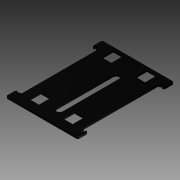
# Autodesk Inventor part: BED ROD MOUNT
Saved by Autodesk Inventor 2013 (Build 170138000, 138)
## iProperties
Created: 2014-03-03
Part Number: BED ROD MOUNT
Material: Generic
Document SubType Name: Modeling
Designer: employee
Density: 1 g/cm^3
Author: employee
Autodesk Inventor part; units mm, degrees
ref_plane "YZ Plane" through (0, 0, 0) normal (1, 0, 0) x (0, 1, 0)
ref_plane "XZ Plane" through (0, 0, 0) normal (0, 1, 0) x (-1, 0, 0)
ref_plane "XY Plane" through (0, 0, 0) normal (0, 0, 1) x (1, 0, 0)
sketch "Sketch1" plane through (0, 0, 0) normal (0, 0, 1) x (1, 0, 0)
  line L0 (-127, 170) -> (127, 170)
  line L1 (127, 170) -> (127, -170)
  line L2 (127, -170) -> (-127, -170)
  line L3 (-127, -170) -> (-127, 170)
  point P0 (0, 0)
  point P1 (0, 170)
  point P2 (-127, 0)
  dimension "d0" = 340
  dimension "d2" = 254
  constraints: 8 end point, 2 midpoint, 2 parallel, 1 horizontal, 1 horizontal alignment, 1 perpendicular, 1 vertical alignment
  measures "d0" distance of L2.end L0.start
  measures "d2" distance of L0.start L0.end
extrude "Extrusion1" add sketch "Sketch1" along normal blind 6.477
sketch "Sketch2" plane through (0, 0, 6.477) normal (0, 0, 1) x (1, 0, 0)
  line L0 (-127, 170) -> (-127, -170) projected
  line L1 (-127, 135) -> (-107, 135)
  line L2 (-107, 135) -> (-107, -135)
  line L3 (-107, -135) -> (-127, -135)
  line L4 (-127, -135) -> (-127, 135)
  point P0 (0, 0)
  point P1 (-127, 0)
  point P2 (-127, 0)
  dimension "d5" = 270
  dimension "d7" = 20
  constraints: 8 end point, 2 midpoint, 2 parallel, 1 coincident, 1 horizontal, 1 perpendicular, 1 point on line
  measures "d5" distance of L1.end L2.end
  measures "d7" distance of L1.start L1.end
extrude "Extrusion2" cut sketch "Sketch2" against normal through all
sketch "Sketch3" plane through (0, 0, 6.477) normal (0, 0, 1) x (1, 0, 0)
  line L0 (-127, 135) -> (-107, 135) projected
  line L1 (-119.8284, 135) -> (-114.1716, 135)
  line L2 (-114.1716, 135) -> (-114.1716, 145)
  line L3 (-114.1716, 145) -> (-119.8284, 145)
  line L4 (-119.8284, 145) -> (-119.8284, 135)
  circle A0 centre (-117, 145) radius 4
  line L5 (-117, 145) -> (-119.8284, 147.8284)
  point P0 (0, 0)
  point P1 (-117, 135)
  point P2 (-117, 135)
  point P3 (-117, 135)
  dimension "d14" = 8
  dimension "d10" = 10
  dimension "d12" = 135
  constraints: 10 end point, 4 midpoint, 2 parallel, 1 coincident, 1 horizontal, 1 perpendicular, 1 point on line, 1 vertical alignment, 3 other
  measures "d10" distance of L3.end L1.start
  measures "d12" angle of L5 L3
extrude "Extrusion3" cut sketch "Sketch3" against normal through all contours L4 A0 L2 L0 | L4 L3 L2 A0
sketch "Sketch4" plane through (0, 0, 6.477) normal (0, 0, 1) x (1, 0, 0)
  line L0 (-119.8284, 135) -> (-119.8284, 145) projected
  line L1 (-119.8284, 145) -> (-114.1716, 145) projected
  line L2 (-121, 142) -> (-113, 142)
  line L3 (-113, 142) -> (-113, 138)
  line L4 (-113, 138) -> (-121, 138)
  line L5 (-121, 138) -> (-121, 142)
  line L6 (-113, 142) -> (-112, 142)
  line L7 (-112, 142) -> (-112, 138)
  line L8 (-112, 138) -> (-113, 138)
  line L9 (-113, 138) -> (-113, 142)
  line L10 (-121, 142) -> (-122, 142)
  line L11 (-122, 142) -> (-122, 138)
  line L12 (-122, 138) -> (-121, 138)
  line L13 (-121, 138) -> (-121, 142)
  point P0 (0, 0)
  point P1 (-117, 142)
  point P2 (-117, 145)
  point P3 (-121, 140)
  point P4 (-119.8284, 140)
  dimension "d17" = 4
  dimension "d19" = 8
  dimension "d20" = 1
  constraints: 24 end point, 6 parallel, 4 midpoint, 3 horizontal, 3 perpendicular, 1 collinear, 1 horizontal alignment, 1 vertical alignment
  measures "d17" distance of L6.end L7.end
  measures "d19" distance between parallel lines of L3 L5
  measures "d20" distance of L2.end L6.end
extrude "Extrusion4" cut sketch "Sketch4" against normal through all contours L3 L6 L7 L8 | L12 L11 L10 L5
fillet "Fillet1" radius 5 2 edges at (-127, 170, 3.2385) (-127, 135, 3.2385)
fillet "Fillet1" radius 2.5 1 edges at (-107, 135, 3.2385)
mirror "Mirror1" about plane through (0, 0, 0) normal (1, 0, 0) of "Extrusion2"
mirror "Mirror2" about plane through (0, 0, 0) normal (1, 0, 0) of "Extrusion4", "Extrusion3", "Fillet1"
mirror "Mirror3" about plane through (0, 0, 0) normal (0, 1, 0) of "Extrusion4", "Extrusion3", "Fillet1", "Mirror2"
sketch "Sketch5" plane through (0, 0, 6.477) normal (0, 0, 1) x (1, 0, 0)
  line L0 (-109.5, -135) -> (-114.1716, -135) projected
  line L1 (-113, 142) -> (-112, 142) projected
  line L2 (20.5, -116.5) -> (20.5, 83.5)
  arc A0 (20.5, 83.5) -> (-1.5, 83.5) centre (9.5, 83.5) ccw
  line L3 (-1.5, 83.5) -> (-1.5, -116.5)
  arc A1 (-1.5, -116.5) -> (20.5, -116.5) centre (9.5, -116.5) ccw
  point P0 (0, 0)
  dimension "d31" = 18.5
  dimension "d32" = 11
  dimension "d33" = 200
  dimension "d34" = 9.5
  constraints: 4 end point, 4 point on circle, 4 tangent, 2 centre point, 1 parallel, 1 perpendicular
  measures "d31" distance from line of A1.centre L0
  measures "d32" radius of A1
  measures "d33" distance of L2.start L2.end
  measures "d34" horizontal distance of A1.centre point (0, 0)
extrude "Extrusion5" cut sketch "Sketch5" against normal through all
sketch "Sketch6" plane through (0, 0, 0) normal (0, 0, -1) x (-1, 0, 0)
  line L0 (-42, 159.6) -> (-77, 159.6) projected
  line L1 (-77, 159.6) -> (-77, 137.6) projected
  line L2 (-77, 137.6) -> (-42, 137.6) projected
  line L3 (-42, 137.6) -> (-42, 159.6) projected
  line L4 (42, -138.4) -> (77, -138.4) projected
  line L5 (77, -138.4) -> (77, -116.4) projected
  line L6 (77, -116.4) -> (42, -116.4) projected
  line L7 (42, -116.4) -> (42, -138.4) projected
  line L8 (-42, -138.4) -> (-42, -116.4) projected
  line L9 (-42, -116.4) -> (-77, -116.4) projected
  line L10 (-77, -116.4) -> (-77, -138.4) projected
  line L11 (-77, -138.4) -> (-42, -138.4) projected
  line L12 (42, 159.6) -> (42, 137.6) projected
  line L13 (42, 137.6) -> (77, 137.6) projected
  line L14 (77, 137.6) -> (77, 159.6) projected
  line L15 (77, 159.6) -> (42, 159.6) projected
  line L16 (101.6, -91) -> (101.6, 112.2) projected
  line L17 (-9.525, 112.2) -> (-101.6, 112.2) projected
  line L18 (-101.6, 112.2) -> (-101.6, -91) projected
  line L19 (-101.6, -91) -> (101.6, -91) projected
  line L20 (112, 138) -> (113, 138) projected
  line L21 (113, 138) -> (113, 142) projected
  line L22 (113, 142) -> (112, 142) projected
  line L23 (112, 142) -> (112, 138) projected
  line L24 (122, 142) -> (121, 142) projected
  line L25 (121, 142) -> (121, 138) projected
  line L26 (121, 138) -> (122, 138) projected
  line L27 (122, 138) -> (122, 142) projected
  line L28 (-121, 142) -> (-122, 142) projected
  line L29 (-122, 142) -> (-122, 138) projected
  line L30 (-122, 138) -> (-121, 138) projected
  line L31 (-121, 138) -> (-121, 142) projected
  line L32 (-113, 142) -> (-113, 138) projected
  line L33 (-113, 138) -> (-112, 138) projected
  line L34 (-112, 138) -> (-112, 142) projected
  line L35 (-112, 142) -> (-113, 142) projected
  line L36 (121, -142) -> (122, -142) projected
  line L37 (122, -142) -> (122, -138) projected
  line L38 (122, -138) -> (121, -138) projected
  line L39 (121, -138) -> (121, -142) projected
  line L40 (113, -142) -> (113, -138) projected
  line L41 (113, -138) -> (112, -138) projected
  line L42 (112, -138) -> (112, -142) projected
  line L43 (112, -142) -> (113, -142) projected
  line L44 (-121, -138) -> (-122, -138) projected
  line L45 (-122, -138) -> (-122, -142) projected
  line L46 (-122, -142) -> (-121, -142) projected
  line L47 (-121, -142) -> (-121, -138) projected
  line L48 (-112, -142) -> (-112, -138) projected
  line L49 (-112, -138) -> (-113, -138) projected
  line L50 (-113, -138) -> (-113, -142) projected
  line L51 (-113, -142) -> (-112, -142) projected
  line L52 (-127, -165) -> (-127, 165) projected
  arc A0 (-122, 170) -> (-127, 165) centre (-122, 165) ccw projected
  line L53 (-122, 170) -> (122, 170) projected
  arc A1 (127, 165) -> (122, 170) centre (122, 165) ccw projected
  line L54 (127, 165) -> (127, -165) projected
  arc A2 (122, -170) -> (127, -165) centre (122, -165) ccw projected
  line L55 (122, -170) -> (-122, -170) projected
  arc A3 (-127, -165) -> (-122, -170) centre (-122, -165) ccw projected
  line L56 (-77, -116.4) -> (-42, -116.4)
  line L57 (-42, -116.4) -> (-42, -96.4)
  line L58 (-42, -96.4) -> (-77, -96.4)
  line L59 (-77, -96.4) -> (-77, -116.4)
  line L60 (42, -116.4) -> (77, -116.4)
  line L61 (77, -116.4) -> (77, -96.4)
  line L62 (77, -96.4) -> (42, -96.4)
  line L63 (42, -96.4) -> (42, -116.4)
  line L64 (-77, 137.6) -> (-42, 137.6)
  line L65 (-42, 137.6) -> (-42, 117.6)
  line L66 (-42, 117.6) -> (-77, 117.6)
  line L67 (-77, 117.6) -> (-77, 137.6)
  line L68 (42, 137.6) -> (77, 137.6)
  line L69 (77, 137.6) -> (77, 117.6)
  line L70 (77, 117.6) -> (42, 117.6)
  line L71 (42, 117.6) -> (42, 137.6)
  circle A4 centre (0, 165) radius 1.25 projected
  circle A5 centre (0, -165) radius 1.25 projected
  circle A6 centre (23, -162.38) radius 5.08 projected
  circle A7 centre (30.6332, -154.7468) radius 0.5 projected
  circle A8 centre (15.3668, -154.7468) radius 0.5 projected
  arc A9 (4.7625, 116.9625) -> (9.525, 112.2) centre (9.525, 116.9625) ccw projected
  line L72 (4.7625, 116.9625) -> (4.7625, 145.5375) projected
  arc A10 (4.7625, 145.5375) -> (-4.7625, 145.5375) centre (0, 145.5375) ccw projected
  line L73 (-4.7625, 145.5375) -> (-4.7625, 116.9625) projected
  arc A11 (-9.525, 112.2) -> (-4.7625, 116.9625) centre (-9.525, 116.9625) ccw projected
  line L74 (101.6, 112.2) -> (9.525, 112.2) projected
  point P0 (0, 0)
  dimension "d35" = 20
  constraints: 32 end point, 8 parallel, 4 horizontal, 4 perpendicular, 3 equal length
  measures "d35" distance of L8.end L57.end
extrude "Extrusion6" cut sketch "Sketch6" against normal through all contours L3 L2 L1 L0 | L65 L66 L67 L2 | L7 L6 L5 L4 | L63 L62 L61 L6 | L11 L10 L9 L8 | L9 L59 L58 L57 | L15 L14 L13 L12 | L13 L69 L70 L71
sketch "Sketch7" plane through (0, 0, 0) normal (0, 0, -1) x (-1, 0, 0)
  line L0 (122, 170) -> (-122, 170) projected
  line L1 (-112, -138) -> (-112, -142) projected
  circle A0 centre (0, 165) radius 1.25
  circle A1 centre (0, -165) radius 1.25
  line L2 (0, -165) -> (0, 165)
  point P0 (0, 0)
  point P1 (0, 0)
  dimension "d38" = 2.5
  dimension "d40" = 5
  constraints: 2 centre point, 2 end point, 2 vertical alignment, 1 coincident, 1 equal radius, 1 midpoint, 1 parallel
  measures "d38" diameter of A0
  measures "d40" distance from line of L0 L2.end
extrude "Extrusion7" cut sketch "Sketch7" against normal through all
sketch "Sketch8" plane through (0, 0, 0) normal (0, 0, -1) x (-1, 0, 0)
  circle A0 centre (23, -162.38) radius 3.175 projected
  point P0 (0, 0)
extrude "Extrusion8" cut sketch "Sketch8" against normal through all
sketch "Sketch9" plane through (0, 0, 0) normal (0, 0, -1) x (-1, 0, 0)
  circle A0 centre (30.6332, -154.7468) radius 0.5 projected
  circle A1 centre (15.3668, -154.7468) radius 0.5 projected
  circle A2 centre (23, -162.38) radius 5.08 projected
  line L0 (15.5, -150) -> (30.5, -150) projected
  line L1 (35.5, -155) -> (35.5, -165) projected
  line L2 (30.5, -170) -> (15.5, -170) projected
  line L3 (10.5, -165) -> (10.5, -155) projected
  arc A3 (35.5, -155) -> (30.5, -150) centre (30.5, -155) ccw projected
  arc A4 (30.5, -170) -> (35.5, -165) centre (30.5, -165) ccw projected
  arc A5 (10.5, -165) -> (15.5, -170) centre (15.5, -165) ccw projected
  arc A6 (15.5, -150) -> (10.5, -155) centre (15.5, -155) ccw projected
  point P0 (0, 0)
extrude "Extrusion9" cut sketch "Sketch9" against normal through all contours A0 | A1
body "Solid1"
